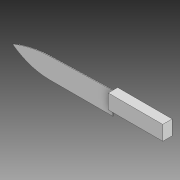
# Autodesk Inventor part: Knife
Saved by Autodesk Inventor 2020 (Build 240168000, 168)
## iProperties
Created: 2020-10-19
Part Number: Knife
Material: Generic
Document SubType Name: Modeling
Designer: DDeGo
Density: 1 g/cm^3
Appearance: Default
Author: DDeGo
Autodesk Inventor part; units mm, degrees
ref_plane "YZ Plane" through (0, 0, 0) normal (1, 0, 0) x (0, 1, 0)
ref_plane "XZ Plane" through (0, 0, 0) normal (0, 1, 0) x (-1, 0, 0)
ref_plane "XY Plane" through (0, 0, 0) normal (0, 0, 1) x (1, 0, 0)
sketch "Sketch1" plane through (0, 0, 0) normal (0, 0, 1) x (1, 0, 0)
  line L0 (0, 0) -> (-100, 0)
  line L1 (-100, 0) -> (-100, 33) construction
  line L2 (-100, 33) -> (0, 36)
  line L3 (0, 36) -> (0, 0)
  arc A0 (-160, 20) -> (-100, 0) centre (-100, 100) ccw
  arc A1 (-100, 33) -> (-160, 20) centre (-94.9522, -135.2589) ccw
  dimension "d0" = 100
  dimension "d2" = 36
  dimension "d10" = 60
  dimension "d11" = 20
  dimension "d12" = 33
  constraints: 8 end point, 4 point on circle, 2 centre point, 2 tangent, 1 horizontal, 1 parallel, 1 perpendicular
  measures "d0" distance between parallel lines of L1 L3
  measures "d2" distance of L2.end L0.start
  measures "d10" distance from line of L1 A0.start
  measures "d11" distance from line of L0 A0.start
  measures "d12" distance of L0.end L1.end
extrude "Extrusion1" add sketch "Sketch1" along normal mid plane 1.1
sketch "Sketch2" plane through (0, 0, 0) normal (0, 0, 1) x (1, 0, 0)
  line L0 (0, 36) -> (-160.3357, 31.1899) projected
  line L1 (0, 36) -> (86.8358, 36)
  line L2 (86.8358, 36) -> (86.8358, 12.7298)
  line L3 (86.8358, 12.7298) -> (0, 12.7298)
  line L4 (0, 12.7298) -> (0, 36)
  point P0 (0, 0)
  point P1 (-160, 20)
  constraints: 8 end point, 2 parallel, 1 horizontal, 1 perpendicular
extrude "Extrusion2" add sketch "Sketch2" along normal mid plane 15
chamfer "Chamfer1" distance 0.5 angle 45 4 edges at (-50, 0, 0.55) (-131.6228, 5.1317, 0.55) (-50, 0, -0.55) (-131.6228, 5.1317, -0.55)
body "Solid1"
